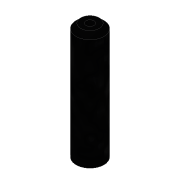
# Autodesk Inventor part: M19 - Wooden Dowel
Saved by Autodesk Inventor 2016 (Build 200138000, 138)
## iProperties
Created: 2017-02-27
Part Number: M19 - Wooden Dowel
Material: Wood (Cherry)
Document SubType Name: Modeling
Designer: Fernando
Stock Number: 0
Mass: 3.21728 g
Surface Area: 25.9231 cm^2
Volume: 5.10679 cm^3
Density: 0.63 g/cm^3
Appearance: Black
SurfaceArea_m2: 0
Author: Fernando
Autodesk Inventor part; units mm, degrees
ref_plane "YZ Plane" through (0, 0, 0) normal (1, 0, 0) x (0, 1, 0)
ref_plane "XZ Plane" through (0, 0, 0) normal (0, 1, 0) x (-1, 0, 0)
ref_plane "XY Plane" through (0, 0, 0) normal (0, 0, 1) x (1, 0, 0)
sketch "Sketch2" plane through (0, 0, 0) normal (0, 0, 1) x (1, 0, 0)
  circle A0 centre (0, 0) radius 6
  circle A1 centre (0, 0) radius 1.75
  dimension "d11" = 12
  dimension "d12" = 3.5
  constraints: 2 centre point, 2 coincident
  measures "d11" diameter of A0
  measures "d12" diameter of A1
extrude "Extrusion2" add sketch "Sketch2" along normal blind 50
chamfer "Chamfer1" distance 2 angle 45 1 edges at (-6, 0, 50)
body "Solid2"
